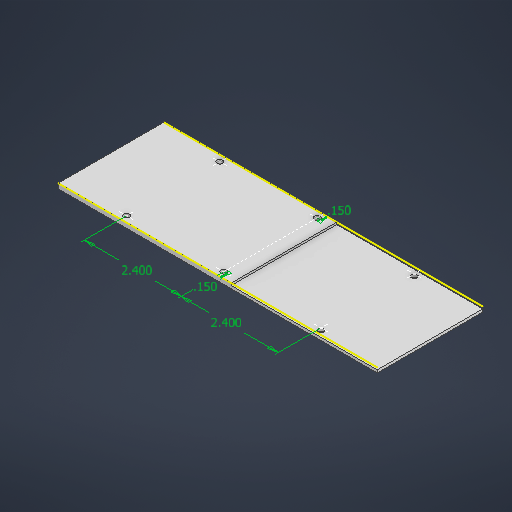
# Autodesk Inventor part: TopLayerPlate
Saved by Autodesk Inventor 2026.2 (Build 302298010, 298A)
## iProperties
Created: 2026-07-14
Part Number: TopLayerPlate
Material: Generic
Document SubType Name: Modeling
Designer: sonata
Density: 1 g/cm^3
Appearance: Default
Author: sonata
Autodesk Inventor part; units mm, degrees
ref_plane "YZ Plane" through (0, 0, 0) normal (1, 0, 0) x (0, 1, 0)
ref_plane "XZ Plane" through (0, 0, 0) normal (0, 1, 0) x (-1, 0, 0)
ref_plane "XY Plane" through (0, 0, 0) normal (0, 0, 1) x (1, 0, 0)
sketch "Sketch1" plane through (0, 0, 0) normal (0, 1, 0) x (-1, 0, 0)
  line L0 (0, 0) -> (200.152, 0)
  line L1 (200.152, 0) -> (200.152, 66.1924)
  line L2 (200.152, 66.1924) -> (0, 66.1924)
  line L3 (0, 66.1924) -> (0, 0)
  dimension "d0" = 66.1924
  dimension "d1" = 200.152
  constraints: 8 end point, 2 parallel, 1 horizontal, 1 perpendicular
  measures "d0" distance of L0.end L1.end
  measures "d1" distance of L1.end L2.end
extrude "Extrusion1" add sketch "Sketch1" along normal blind 3.048
sketch "Sketch2" plane through (0, 3.048, 0) normal (0, 1, 0) x (1, 0, 0)
  line L0 (-200.152, -66.1924) -> (0, -66.1924) projected
  line L1 (-100.076, -66.1924) -> (-100.076, 0) construction
  line L2 (0, 0) -> (-200.152, 0) projected
  point P0 (-100.076, -62.3824)
  point P1 (-100.076, -3.81)
  point P2 (-39.116, -62.3824)
  point P3 (-39.116, -3.81)
  point P4 (-161.036, -3.81)
  point P5 (-161.036, -62.3824)
  dimension "d4" = 3.81
  dimension "d5" = 3.81
  dimension "d6" = 60.96
  dimension "d7" = 60.96
  constraints: 4 horizontal alignment, 2 end point, 2 midpoint, 2 point on line, 2 vertical alignment
  measures "d4" distance from line of L0 point (-100.076, -62.382)
  measures "d5" distance from line of L2 point (-100.076, -3.81)
  measures "d6" distance of point (-100.076, -62.382) point (-161.036, -62.382)
  measures "d7" distance of point (-39.116, -62.382) point (-100.076, -62.382)
hole "Hole1" at (-100.076, 3.048, 62.3824) at (-100.076, 3.048, 3.81) at (-39.116, 3.048, 62.3824) at (-39.116, 3.048, 3.81) at (-161.036, 3.048, 3.81) at (-161.036, 3.048, 62.3824) direction (0, -1, 0) diameter 3.6576 end through all
sketch "Sketch3" plane through (0, 3.048, 0) normal (0, 1, 0) x (1, 0, 0)
  line L0 (0, -66.1924) -> (0, 0) projected
  line L1 (0, -66.1924) -> (-91.6178, -66.1924)
  line L2 (-91.6178, -66.1924) -> (-91.6178, 0)
  line L3 (-91.6178, 0) -> (0, 0)
  line L4 (0, 0) -> (0, -66.1924)
  line L5 (0, 0) -> (-200.152, 0) projected
  point P0 (-100.076, 0)
  dimension "d15" = 8.4582
  constraints: 8 end point, 2 parallel, 1 collinear, 1 horizontal, 1 midpoint, 1 perpendicular
  measures "d15" distance from line of point (-100.076, 0) L2
extrude "Extrusion2" cut sketch "Sketch3" against normal blind 1.3208
body "Solid1"
